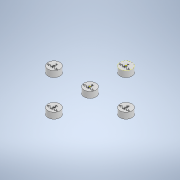
# Autodesk Inventor part: 5-circles-test-print
Saved by Autodesk Inventor 2020.3 (Build 243373000, 373)
## iProperties
Created: 2020-06-02
Part Number: 5-circles-test-print
Material: Generic
Document SubType Name: Modeling
Designer: robst
Density: 1 g/cm^3
Appearance: Default
Author: robst
Autodesk Inventor part; units mm, degrees
ref_plane "YZ Plane" through (0, 0, 0) normal (1, 0, 0) x (0, 1, 0)
ref_plane "XZ Plane" through (0, 0, 0) normal (0, 1, 0) x (-1, 0, 0)
ref_plane "XY Plane" through (0, 0, 0) normal (0, 0, 1) x (1, 0, 0)
sketch "Sketch1" plane through (0, 0, 0) normal (0, 1, 0) x (-1, 0, 0)
  circle A0 centre (0, 0) radius 12.7
  circle A1 centre (76.2, 0) radius 12.7
  circle A2 centre (0, -76.2) radius 12.7
  circle A3 centre (-76.2, 0) radius 12.7
  circle A4 centre (0, 76.2) radius 12.7
  dimension "d0" = 25.4
  dimension "d1" = 76.2
  dimension "d2" = 76.2
  dimension "d3" = 76.2
  dimension "d4" = 76.2
  constraints: 5 centre point, 4 equal radius, 1 coincident
  measures "d0" diameter of A0
  measures "d1" distance of A1.centre point (0, 0)
  measures "d2" distance of A2.centre point (0, 0)
  measures "d3" distance of A3.centre point (0, 0)
  measures "d4" distance of A4.centre point (0, 0)
extrude "Extrusion1" add sketch "Sketch1" along normal blind 12.7
sketch "Sketch4" plane through (0, 12.7, -76.2) normal (0, 1, 0) x (1, 0, 0)
  circle A0 centre (0, 0) radius 12.7 construction
  point P0 (0, -76.2)
sketch "Sketch5" plane through (0, 12.7, 0) normal (0, 1, 0) x (1, 0, 0)
  circle A0 centre (0, 76.2) radius 12.7 construction
  line L0 (-12.7, 76.2) -> (12.7, 76.2) construction
  circle A1 centre (0, 0) radius 12.7 construction
  line L1 (-12.7, 0) -> (12.7, 0) construction
  line L2 (-88.5573, 0) -> (-63.5, 0) construction
  circle A2 centre (-76.2, 0) radius 12.7 construction
  circle A3 centre (76.2, 0) radius 12.7 construction
  line L3 (63.5, 0) -> (88.9, 0) construction
  circle A4 centre (0, -76.2) radius 12.7 construction
  line L4 (-12.7, -76.2) -> (12.7, -76.2) construction
  line L5 (1.6105, 76.2) -> (-1.3634, 76.2)
  line L6 (-1.3634, 76.2) -> (-1.3634, 76.8224)
  line L7 (-1.3634, 76.8224) -> (-0.2569, 76.8224)
  line L8 (-0.2569, 76.8224) -> (-0.2569, 80.9079)
  line L9 (-0.2569, 80.9079) -> (-1.3634, 80.9079)
  line L10 (-1.3634, 80.9079) -> (-1.3634, 81.4661)
  spline S0 degree 2 poles (-1.3634, 81.4661) (-0.7361, 81.4661) (-0.1433, 81.8218) (-0.1037, 82.3158) knots 0 0 0 1 2 2 2
  line L11 (-0.1037, 82.3158) -> (0.5286, 82.3158)
  line L12 (0.5286, 82.3158) -> (0.5286, 76.8224)
  line L13 (0.5286, 76.8224) -> (1.6105, 76.8224)
  line L14 (1.6105, 76.8224) -> (1.6105, 76.2)
  line L15 (-6.3554, 70.4251) -> (-10.752, 72.5246)
  line L16 (-10.752, 72.5246) -> (-10.752, 73.0137)
  line L17 (-10.752, 73.0137) -> (-6.3554, 75.1132)
  line L18 (-6.3554, 75.1132) -> (-6.3554, 74.387)
  line L19 (-6.3554, 74.387) -> (-9.764, 72.7716)
  line L20 (-9.764, 72.7716) -> (-6.3554, 71.1513)
  line L21 (-6.3554, 71.1513) -> (-6.3554, 70.4251)
  line L22 (-2.7985, 72.4011) -> (-5.1055, 72.4011)
  line L23 (-5.1055, 72.4011) -> (-5.1055, 73.1421)
  line L24 (-5.1055, 73.1421) -> (-2.7985, 73.1421)
  line L25 (-2.7985, 73.1421) -> (-2.7985, 72.4011)
  line L26 (2.3984, 70.104) -> (1.4697, 70.104)
  line L27 (1.4697, 70.104) -> (-0.0124, 72.5345)
  line L28 (-0.0124, 72.5345) -> (-1.524, 70.104)
  line L29 (-1.524, 70.104) -> (-2.3984, 70.104)
  line L30 (-2.3984, 70.104) -> (-0.457, 73.1569)
  line L31 (-0.457, 73.1569) -> (-2.3391, 76.2)
  line L32 (-2.3391, 76.2) -> (-1.4104, 76.2)
  line L33 (-1.4104, 76.2) -> (0.042, 73.814)
  line L34 (0.042, 73.814) -> (1.524, 76.2)
  line L35 (1.524, 76.2) -> (2.3984, 76.2)
  line L36 (2.3984, 76.2) -> (0.4915, 73.1965)
  line L37 (0.4915, 73.1965) -> (2.3984, 70.104)
  line L38 (5.1105, 72.4011) -> (2.8035, 72.4011)
  line L39 (2.8035, 72.4011) -> (2.8035, 73.1421)
  line L40 (2.8035, 73.1421) -> (5.1105, 73.1421)
  line L41 (5.1105, 73.1421) -> (5.1105, 72.4011)
  line L42 (10.752, 72.5246) -> (6.3554, 70.4251)
  line L43 (6.3554, 70.4251) -> (6.3554, 71.1513)
  line L44 (6.3554, 71.1513) -> (9.764, 72.7716)
  line L45 (9.764, 72.7716) -> (6.3554, 74.387)
  line L46 (6.3554, 74.387) -> (6.3554, 75.1132)
  line L47 (6.3554, 75.1132) -> (10.752, 73.0137)
  line L48 (10.752, 73.0137) -> (10.752, 72.5246)
  line L49 (-74.1119, 0) -> (-77.8713, 0)
  line L50 (-77.8713, 0) -> (-77.8713, 0.8645)
  spline S1 degree 2 poles (-77.8713, 0.8645) (-77.4662, 1.2449) (-76.7449, 1.9513) (-76.3991, 2.3317) knots 0 0 0 1 2 2 2
  spline S2 degree 2 poles (-76.3991, 2.3317) (-75.7026, 3.0974) (-75.1938, 4.0162) (-75.1938, 4.5053) knots 0 0 0 1 2 2 2
  spline S3 degree 2 poles (-75.1938, 4.5053) (-75.1938, 4.7622) (-75.3519, 5.1475) (-75.4951, 5.271) knots 0 0 0 1 2 2 2
  spline S4 degree 2 poles (-75.4951, 5.271) (-75.6384, 5.3945) (-76.0138, 5.518) (-76.2411, 5.518) knots 0 0 0 1 2 2 2
  spline S5 degree 2 poles (-76.2411, 5.518) (-76.4584, 5.518) (-76.903, 5.4093) (-77.1056, 5.3254) knots 0 0 0 1 2 2 2
  spline S6 degree 2 poles (-77.1056, 5.3254) (-77.2785, 5.2562) (-77.5996, 5.0586) (-77.6984, 4.9894) knots 0 0 0 1 2 2 2
  line L51 (-77.6984, 4.9894) -> (-77.7428, 4.9894)
  line L52 (-77.7428, 4.9894) -> (-77.7428, 5.8589)
  spline S7 degree 2 poles (-77.7428, 5.8589) (-77.4909, 5.9824) (-76.5869, 6.2244) (-76.1818, 6.2244) knots 0 0 0 1 2 2 2
  spline S8 degree 2 poles (-76.1818, 6.2244) (-75.3272, 6.2244) (-74.3639, 5.3204) (-74.3639, 4.5498) knots 0 0 0 1 2 2 2
  spline S9 degree 2 poles (-74.3639, 4.5498) (-74.3639, 4.1891) (-74.5318, 3.5865) (-74.68, 3.3296) knots 0 0 0 1 2 2 2
  spline S10 degree 2 poles (-74.68, 3.3296) (-74.8282, 3.0628) (-75.258, 2.5392) (-75.4951, 2.2872) knots 0 0 0 1 2 2 2
  spline S11 degree 2 poles (-75.4951, 2.2872) (-75.8804, 1.8673) (-76.824, 0.9682) (-77.1056, 0.7064) knots 0 0 0 1 2 2 2
  line L53 (-77.1056, 0.7064) -> (-74.1119, 0.7064)
  line L54 (-74.1119, 0.7064) -> (-74.1119, 0)
  line L55 (-82.384, -5.7749) -> (-86.7806, -3.6754)
  line L56 (-86.7806, -3.6754) -> (-86.7806, -3.1863)
  line L57 (-86.7806, -3.1863) -> (-82.384, -1.0868)
  line L58 (-82.384, -1.0868) -> (-82.384, -1.813)
  line L59 (-82.384, -1.813) -> (-85.7926, -3.4284)
  line L60 (-85.7926, -3.4284) -> (-82.384, -5.0487)
  line L61 (-82.384, -5.0487) -> (-82.384, -5.7749)
  line L62 (-78.8272, -3.7989) -> (-81.1342, -3.7989)
  line L63 (-81.1342, -3.7989) -> (-81.1342, -3.0579)
  line L64 (-81.1342, -3.0579) -> (-78.8272, -3.0579)
  line L65 (-78.8272, -3.0579) -> (-78.8272, -3.7989)
  line L66 (-73.6303, -6.096) -> (-74.559, -6.096)
  line L67 (-74.559, -6.096) -> (-76.041, -3.6655)
  line L68 (-76.041, -3.6655) -> (-77.5526, -6.096)
  line L69 (-77.5526, -6.096) -> (-78.427, -6.096)
  line L70 (-78.427, -6.096) -> (-76.4856, -3.0431)
  line L71 (-76.4856, -3.0431) -> (-78.3677, 0)
  line L72 (-78.3677, 0) -> (-77.439, 0)
  line L73 (-77.439, 0) -> (-75.9867, -2.386)
  line L74 (-75.9867, -2.386) -> (-74.5046, 0)
  line L75 (-74.5046, 0) -> (-73.6303, 0)
  line L76 (-73.6303, 0) -> (-75.5371, -3.0035)
  line L77 (-75.5371, -3.0035) -> (-73.6303, -6.096)
  line L78 (-70.9182, -3.7989) -> (-73.2252, -3.7989)
  line L79 (-73.2252, -3.7989) -> (-73.2252, -3.0579)
  line L80 (-73.2252, -3.0579) -> (-70.9182, -3.0579)
  line L81 (-70.9182, -3.0579) -> (-70.9182, -3.7989)
  line L82 (-65.2767, -3.6754) -> (-69.6733, -5.7749)
  line L83 (-69.6733, -5.7749) -> (-69.6733, -5.0487)
  line L84 (-69.6733, -5.0487) -> (-66.2647, -3.4284)
  line L85 (-66.2647, -3.4284) -> (-69.6733, -1.813)
  line L86 (-69.6733, -1.813) -> (-69.6733, -1.0868)
  line L87 (-69.6733, -1.0868) -> (-65.2767, -3.1863)
  line L88 (-65.2767, -3.1863) -> (-65.2767, -3.6754)
  spline S12 degree 2 poles (-0.1976, 5.518) (-0.4199, 5.518) (-0.8596, 5.4093) (-1.072, 5.3254) knots 0 0 0 1 2 2 2
  spline S13 degree 2 poles (-1.072, 5.3254) (-1.2696, 5.2414) (-1.5611, 5.0635) (-1.6747, 4.9845) knots 0 0 0 1 2 2 2
  line L89 (-1.6747, 4.9845) -> (-1.7241, 4.9845)
  line L90 (-1.7241, 4.9845) -> (-1.7241, 5.849)
  spline S14 degree 2 poles (-1.7241, 5.849) (-1.4573, 5.9923) (-0.5434, 6.2244) (-0.1334, 6.2244) knots 0 0 0 1 2 2 2
  spline S15 degree 2 poles (-0.1334, 6.2244) (0.2816, 6.2244) (0.8991, 6.0565) (1.151, 5.8786) knots 0 0 0 1 2 2 2
  spline S16 degree 2 poles (1.151, 5.8786) (1.4178, 5.686) (1.6944, 5.1278) (1.6944, 4.7523) knots 0 0 0 1 2 2 2
  spline S17 degree 2 poles (1.6944, 4.7523) (1.6944, 4.2484) (1.0325, 3.4877) (0.5681, 3.3889) knots 0 0 0 1 2 2 2
  line L91 (0.5681, 3.3889) -> (0.5681, 3.3296)
  spline S18 degree 2 poles (0.5681, 3.3296) (0.7608, 3.2901) (1.2004, 3.1122) (1.3881, 2.9344) knots 0 0 0 1 2 2 2
  spline S19 degree 2 poles (1.3881, 2.9344) (1.5759, 2.7615) (1.813, 2.2082) (1.813, 1.8081) knots 0 0 0 1 2 2 2
  spline S20 degree 2 poles (1.813, 1.8081) (1.813, 1.398) (1.5314, 0.7015) (1.2745, 0.4347) knots 0 0 0 1 2 2 2
  spline S21 degree 2 poles (1.2745, 0.4347) (1.0078, 0.1581) (0.2519, -0.1284) (-0.2272, -0.1284) knots 0 0 0 1 2 2 2
  spline S22 degree 2 poles (-0.2272, -0.1284) (-0.6867, -0.1284) (-1.5858, 0.0939) (-1.892, 0.247) knots 0 0 0 1 2 2 2
  line L92 (-1.892, 0.247) -> (-1.892, 1.1115)
  line L93 (-1.892, 1.1115) -> (-1.8328, 1.1115)
  spline S23 degree 2 poles (-1.8328, 1.1115) (-1.5759, 0.9238) (-0.7064, 0.578) (-0.2766, 0.578) knots 0 0 0 1 2 2 2
  spline S24 degree 2 poles (-0.2766, 0.578) (-0.0247, 0.578) (0.4792, 0.7361) (0.6471, 0.9188) knots 0 0 0 1 2 2 2
  spline S25 degree 2 poles (0.6471, 0.9188) (0.8102, 1.1016) (0.9831, 1.5364) (0.9831, 1.8673) knots 0 0 0 1 2 2 2
  spline S26 degree 2 poles (0.9831, 1.8673) (0.9831, 2.1983) (0.7904, 2.6281) (0.6175, 2.7516) knots 0 0 0 1 2 2 2
  spline S27 degree 2 poles (0.6175, 2.7516) (0.4446, 2.8751) (-0.0247, 2.969) (-0.3013, 2.969) knots 0 0 0 1 2 2 2
  line L94 (-0.3013, 2.969) -> (-0.6471, 2.969)
  line L95 (-0.6471, 2.969) -> (-0.6471, 3.6457)
  line L96 (-0.6471, 3.6457) -> (-0.3754, 3.6457)
  spline S28 degree 2 poles (-0.3754, 3.6457) (0.1729, 3.6457) (0.8645, 4.1694) (0.8645, 4.6683) knots 0 0 0 1 2 2 2
  spline S29 degree 2 poles (0.8645, 4.6683) (0.8645, 4.9005) (0.6867, 5.2315) (0.5434, 5.3303) knots 0 0 0 1 2 2 2
  spline S30 degree 2 poles (0.5434, 5.3303) (0.3903, 5.434) (0.0148, 5.518) (-0.1976, 5.518) knots 0 0 0 1 2 2 2
  line L97 (-6.3554, -5.7749) -> (-10.752, -3.6754)
  line L98 (-10.752, -3.6754) -> (-10.752, -3.1863)
  line L99 (-10.752, -3.1863) -> (-6.3554, -1.0868)
  line L100 (-6.3554, -1.0868) -> (-6.3554, -1.813)
  line L101 (-6.3554, -1.813) -> (-9.764, -3.4284)
  line L102 (-9.764, -3.4284) -> (-6.3554, -5.0487)
  line L103 (-6.3554, -5.0487) -> (-6.3554, -5.7749)
  line L104 (-2.7985, -3.7989) -> (-5.1055, -3.7989)
  line L105 (-5.1055, -3.7989) -> (-5.1055, -3.0579)
  line L106 (-5.1055, -3.0579) -> (-2.7985, -3.0579)
  line L107 (-2.7985, -3.0579) -> (-2.7985, -3.7989)
  line L108 (2.3984, -6.096) -> (1.4697, -6.096)
  line L109 (1.4697, -6.096) -> (-0.0124, -3.6655)
  line L110 (-0.0124, -3.6655) -> (-1.524, -6.096)
  line L111 (-1.524, -6.096) -> (-2.3984, -6.096)
  line L112 (-2.3984, -6.096) -> (-0.457, -3.0431)
  line L113 (-0.457, -3.0431) -> (-2.3391, 0)
  line L114 (-2.3391, 0) -> (-1.4104, 0)
  line L115 (-1.4104, 0) -> (0.042, -2.386)
  line L116 (0.042, -2.386) -> (1.524, 0)
  line L117 (1.524, 0) -> (2.3984, 0)
  line L118 (2.3984, 0) -> (0.4915, -3.0035)
  line L119 (0.4915, -3.0035) -> (2.3984, -6.096)
  line L120 (5.1105, -3.7989) -> (2.8035, -3.7989)
  line L121 (2.8035, -3.7989) -> (2.8035, -3.0579)
  line L122 (2.8035, -3.0579) -> (5.1105, -3.0579)
  line L123 (5.1105, -3.0579) -> (5.1105, -3.7989)
  line L124 (10.752, -3.6754) -> (6.3554, -5.7749)
  line L125 (6.3554, -5.7749) -> (6.3554, -5.0487)
  line L126 (6.3554, -5.0487) -> (9.764, -3.4284)
  line L127 (9.764, -3.4284) -> (6.3554, -1.813)
  line L128 (6.3554, -1.813) -> (6.3554, -1.0868)
  line L129 (6.3554, -1.0868) -> (10.752, -3.1863)
  line L130 (10.752, -3.1863) -> (10.752, -3.6754)
  line L131 (78.2798, 2.0946) -> (77.5536, 2.0946)
  line L132 (77.5536, 2.0946) -> (77.5536, 0)
  line L133 (77.5536, 0) -> (76.7681, 0)
  line L134 (76.7681, 0) -> (76.7681, 2.0946)
  line L135 (76.7681, 2.0946) -> (74.0758, 2.0946)
  line L136 (74.0758, 2.0946) -> (74.0758, 2.9541)
  line L137 (74.0758, 2.9541) -> (76.8027, 6.096)
  line L138 (76.8027, 6.096) -> (77.5536, 6.096)
  line L139 (77.5536, 6.096) -> (77.5536, 2.7516)
  line L140 (77.5536, 2.7516) -> (78.2798, 2.7516)
  line L141 (78.2798, 2.7516) -> (78.2798, 2.0946)
  line L142 (76.7681, 2.7516) -> (76.7681, 5.1327)
  line L143 (76.7681, 5.1327) -> (74.718, 2.7516)
  line L144 (74.718, 2.7516) -> (76.7681, 2.7516)
  line L145 (69.8446, -5.7749) -> (65.448, -3.6754)
  line L146 (65.448, -3.6754) -> (65.448, -3.1863)
  line L147 (65.448, -3.1863) -> (69.8446, -1.0868)
  line L148 (69.8446, -1.0868) -> (69.8446, -1.813)
  line L149 (69.8446, -1.813) -> (66.436, -3.4284)
  line L150 (66.436, -3.4284) -> (69.8446, -5.0487)
  line L151 (69.8446, -5.0487) -> (69.8446, -5.7749)
  line L152 (73.4015, -3.7989) -> (71.0945, -3.7989)
  line L153 (71.0945, -3.7989) -> (71.0945, -3.0579)
  line L154 (71.0945, -3.0579) -> (73.4015, -3.0579)
  line L155 (73.4015, -3.0579) -> (73.4015, -3.7989)
  line L156 (78.5984, -6.096) -> (77.6697, -6.096)
  line L157 (77.6697, -6.096) -> (76.1876, -3.6655)
  line L158 (76.1876, -3.6655) -> (74.676, -6.096)
  line L159 (74.676, -6.096) -> (73.8016, -6.096)
  line L160 (73.8016, -6.096) -> (75.743, -3.0431)
  line L161 (75.743, -3.0431) -> (73.8609, 0)
  line L162 (73.8609, 0) -> (74.7896, 0)
  line L163 (74.7896, 0) -> (76.242, -2.386)
  line L164 (76.242, -2.386) -> (77.724, 0)
  line L165 (77.724, 0) -> (78.5984, 0)
  line L166 (78.5984, 0) -> (76.6915, -3.0035)
  line L167 (76.6915, -3.0035) -> (78.5984, -6.096)
  line L168 (81.3105, -3.7989) -> (79.0035, -3.7989)
  line L169 (79.0035, -3.7989) -> (79.0035, -3.0579)
  line L170 (79.0035, -3.0579) -> (81.3105, -3.0579)
  line L171 (81.3105, -3.0579) -> (81.3105, -3.7989)
  line L172 (86.952, -3.6754) -> (82.5554, -5.7749)
  line L173 (82.5554, -5.7749) -> (82.5554, -5.0487)
  line L174 (82.5554, -5.0487) -> (85.964, -3.4284)
  line L175 (85.964, -3.4284) -> (82.5554, -1.813)
  line L176 (82.5554, -1.813) -> (82.5554, -1.0868)
  line L177 (82.5554, -1.0868) -> (86.952, -3.1863)
  line L178 (86.952, -3.1863) -> (86.952, -3.6754)
  spline S31 degree 2 poles (1.8525, -74.2635) (1.8525, -74.7032) (1.5709, -75.4541) (1.314, -75.7307) knots 0 0 0 1 2 2 2
  spline S32 degree 2 poles (1.314, -75.7307) (1.0572, -76.0073) (0.2915, -76.3284) (-0.1828, -76.3284) knots 0 0 0 1 2 2 2
  spline S33 degree 2 poles (-0.1828, -76.3284) (-0.6175, -76.3284) (-1.4672, -76.1358) (-1.7784, -75.9826) knots 0 0 0 1 2 2 2
  line L179 (-1.7784, -75.9826) -> (-1.7784, -75.1181)
  line L180 (-1.7784, -75.1181) -> (-1.7191, -75.1181)
  spline S34 degree 2 poles (-1.7191, -75.1181) (-1.6253, -75.1873) (-1.2745, -75.3651) (-1.0621, -75.4442) knots 0 0 0 1 2 2 2
  spline S35 degree 2 poles (-1.0621, -75.4442) (-0.82, -75.5282) (-0.4199, -75.622) (-0.168, -75.622) knots 0 0 0 1 2 2 2
  spline S36 degree 2 poles (-0.168, -75.622) (0.079, -75.622) (0.5434, -75.4442) (0.7114, -75.2515) knots 0 0 0 1 2 2 2
  spline S37 degree 2 poles (0.7114, -75.2515) (0.8645, -75.0687) (1.0226, -74.5846) (1.0226, -74.2586) knots 0 0 0 1 2 2 2
  spline S38 degree 2 poles (1.0226, -74.2586) (1.0226, -73.9325) (0.8447, -73.5176) (0.6768, -73.3792) knots 0 0 0 1 2 2 2
  spline S39 degree 2 poles (0.6768, -73.3792) (0.5039, -73.2261) (-0.0099, -73.0977) (-0.3211, -73.0977) knots 0 0 0 1 2 2 2
  spline S40 degree 2 poles (-0.3211, -73.0977) (-0.657, -73.0977) (-1.3239, -73.2014) (-1.5265, -73.2459) knots 0 0 0 1 2 2 2
  line L181 (-1.5265, -73.2459) -> (-1.5265, -70.104)
  line L182 (-1.5265, -70.104) -> (1.8179, -70.104)
  line L183 (1.8179, -70.104) -> (1.8179, -70.8203)
  line L184 (1.8179, -70.8203) -> (-0.741, -70.8203)
  line L185 (-0.741, -70.8203) -> (-0.741, -72.4456)
  spline S41 degree 2 poles (-0.741, -72.4456) (-0.5928, -72.4258) (-0.3063, -72.411) (-0.1877, -72.411) knots 0 0 0 1 2 2 2
  spline S42 degree 2 poles (-0.1877, -72.411) (0.2816, -72.411) (0.9287, -72.5641) (1.2251, -72.7914) knots 0 0 0 1 2 2 2
  spline S43 degree 2 poles (1.2251, -72.7914) (1.5265, -73.0186) (1.8525, -73.7102) (1.8525, -74.2635) knots 0 0 0 1 2 2 2
  line L186 (-6.3554, -81.9749) -> (-10.752, -79.8754)
  line L187 (-10.752, -79.8754) -> (-10.752, -79.3863)
  line L188 (-10.752, -79.3863) -> (-6.3554, -77.2868)
  line L189 (-6.3554, -77.2868) -> (-6.3554, -78.013)
  line L190 (-6.3554, -78.013) -> (-9.764, -79.6284)
  line L191 (-9.764, -79.6284) -> (-6.3554, -81.2487)
  line L192 (-6.3554, -81.2487) -> (-6.3554, -81.9749)
  line L193 (-2.7985, -79.9989) -> (-5.1055, -79.9989)
  line L194 (-5.1055, -79.9989) -> (-5.1055, -79.2579)
  line L195 (-5.1055, -79.2579) -> (-2.7985, -79.2579)
  line L196 (-2.7985, -79.2579) -> (-2.7985, -79.9989)
  line L197 (2.3984, -82.296) -> (1.4697, -82.296)
  line L198 (1.4697, -82.296) -> (-0.0124, -79.8655)
  line L199 (-0.0124, -79.8655) -> (-1.524, -82.296)
  line L200 (-1.524, -82.296) -> (-2.3984, -82.296)
  line L201 (-2.3984, -82.296) -> (-0.457, -79.2431)
  line L202 (-0.457, -79.2431) -> (-2.3391, -76.2)
  line L203 (-2.3391, -76.2) -> (-1.4104, -76.2)
  line L204 (-1.4104, -76.2) -> (0.042, -78.586)
  line L205 (0.042, -78.586) -> (1.524, -76.2)
  line L206 (1.524, -76.2) -> (2.3984, -76.2)
  line L207 (2.3984, -76.2) -> (0.4915, -79.2035)
  line L208 (0.4915, -79.2035) -> (2.3984, -82.296)
  line L209 (5.1105, -79.9989) -> (2.8035, -79.9989)
  line L210 (2.8035, -79.9989) -> (2.8035, -79.2579)
  line L211 (2.8035, -79.2579) -> (5.1105, -79.2579)
  line L212 (5.1105, -79.2579) -> (5.1105, -79.9989)
  line L213 (10.752, -79.8754) -> (6.3554, -81.9749)
  line L214 (6.3554, -81.9749) -> (6.3554, -81.2487)
  line L215 (6.3554, -81.2487) -> (9.764, -79.6284)
  line L216 (9.764, -79.6284) -> (6.3554, -78.013)
  line L217 (6.3554, -78.013) -> (6.3554, -77.2868)
  line L218 (6.3554, -77.2868) -> (10.752, -79.3863)
  line L219 (10.752, -79.3863) -> (10.752, -79.8754)
  constraints: 12 horizontal, 10 end point, 8 point on circle, 2 point on line, 1 horizontal alignment, 1 parallel, 1 other
extrude "Extrusion4" cut sketch "Sketch5" against normal blind 2.54 contours L35 L36 L37 L26 L27 L28 L29 L30 L31 L32 L33 L34 L5 | L5 L6 L7 L8 L9 L10 S0 L11 L12 L13 L14 | L15 L16 L17 L18 L19 L20 L21 | L22 L23 L24 L25 | L38 L39 L40 L41 | L42 L43 L44 L45 L46 L47 L48 | L75 L76 L77 L66 L67 L68 L69 L70 L71 L72 L49 L73 L74 | L49 L50 S1 S2 S3 S4 S5 S6 L51 L52 S7 S8 S9 S10 S11 L53 L54 | L55 L56 L57 L58 L59 L60 L61 | L62 L63 L64 L65 | L78 L79 L80 L81 | L82 L83 L84 L85 L86 L87 L88 | S12 S13 L89 L90 S14 S15 S16 S17 L91 S18 S19 S20 S21 S22 L92 L93 S23 S24 S25 S26 S27 L94 L95 L96 S28 S29 S30 | L97 L98 L99 L100 L101 L102 L103 | L104 L105 L106 L107 | L108 L109 L110 L111 L112 L113 L114 L115 L116 L117 L118 L119 | L120 L121 L122 L123 | L124 L125 L126 L127 L128 L129 L130 | L131 L132 L133 L134 L135 L136 L137 L138 L139 L140 L141 | L145 L146 L147 L148 L149 L150 L151 | L152 L153 L154 L155 | L156 L157 L158 L159 L160 L161 L162 L163 L164 L165 L166 L167 | L168 L169 L170 L171 | L172 L173 L174 L175 L176 L177 L178 | S31 S32 S33 L179 L180 S34 S35 S36 S37 S38 S39 S40 L181 L182 L183 L184 L185 S41 S42 S43 | L186 L187 L188 L189 L190 L191 L192 | L193 L194 L195 L196 | L197 L198 L199 L200 L201 L202 L203 L204 L205 L206 L207 L208 | L209 L210 L211 L212 | L213 L214 L215 L216 L217 L218 L219
body "Solid1"
